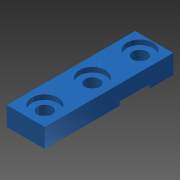
# Autodesk Inventor part: XCarriageBeltClampRight
Saved by Autodesk Inventor 2015 (Build 190159000, 159)
## iProperties
Created: 2014-08-22
Part Number: XCarriageBeltClampRight
Material: ABS Plastic
Document SubType Name: Modeling
Designer: t_clevj
Density: 1.06 g/cm^3
Appearance: Cyan
Author: t_clevj
Autodesk Inventor part; units mm, degrees
ref_plane "YZ Plane" through (0, 0, 0) normal (1, 0, 0) x (0, 1, 0)
ref_plane "XZ Plane" through (0, 0, 0) normal (0, 1, 0) x (-1, 0, 0)
ref_plane "XY Plane" through (0, 0, 0) normal (0, 0, 1) x (1, 0, 0)
sketch "Sketch1" plane through (0, 0, 0) normal (0, 0, 1) x (1, 0, 0)
  line L0 (0, 0) -> (8, 0)
  line L1 (8, 0) -> (8, 27)
  line L2 (8, 27) -> (0, 27)
  line L3 (0, 27) -> (0, 0)
  dimension "d0" = 27
  dimension "d1" = 8
  constraints: 8 end point, 2 parallel, 1 horizontal, 1 perpendicular
  measures "d0" distance of L2.end L0.start
  measures "d1" distance of L0.start L0.end
extrude "Extrusion1" add sketch "Sketch1" along normal blind 4
sketch "Sketch2" plane through (0, 0, 4) normal (0, 0, 1) x (1, 0, 0)
  line L0 (8, 0) -> (8, 27) projected
  line L1 (8, 27) -> (0, 27) projected
  point P0 (4, 24)
  point P1 (4, 14)
  point P2 (4, 4)
  dimension "d5" = 20
  dimension "d6" = 10
  dimension "d7" = 4
  dimension "d15" = 3
  constraints: 2 vertical alignment
  measures "d5" distance of point (4, 24) point (4, 4)
  measures "d6" distance of point (4, 4) point (4, 14)
  measures "d7" distance from line of L0 point (4, 4)
  measures "d15" distance from line of L1 point (4, 24)
hole "Hole1" at (4, 24, 4) at (4, 14, 4) at (4, 4, 4) direction (0, 0, -1) diameter 3 end up to face face through (2.6667, 18, 0) facing (0, 0, -1) counterbore diameter 5.5 counterbore depth 1
sketch "Sketch3" plane through (0, 0, 0) normal (0, 0, -1) x (-1, 0, 0)
  circle A0 centre (-4, 14) radius 1.5 projected
  line L0 (0, 27) -> (0, 0) projected
  line L1 (-8, 0) -> (-8, 27) projected
  line L2 (0, 27) -> (0, 0) construction
  line L3 (0, 22.25) -> (-8, 22.25) construction
  line L4 (-8, 0) -> (-8, 27) construction
  line L5 (-8, 15.75) -> (0, 15.75) construction
  line L6 (-8, 22.25) -> (-6.7, 22.25)
  line L7 (-6.7, 22.25) -> (-6.7, 15.75)
  line L8 (-6.7, 15.75) -> (-8, 15.75)
  line L9 (-8, 15.75) -> (-8, 22.25)
  line L10 (-6, 15.75) -> (-4.7, 15.75)
  line L11 (-4.7, 15.75) -> (-4.7, 22.25)
  line L12 (-4.7, 22.25) -> (-6, 22.25)
  line L13 (-6, 22.25) -> (-6, 15.75)
  line L14 (-4, 15.75) -> (-2.7, 15.75)
  line L15 (-2.7, 15.75) -> (-2.7, 22.25)
  line L16 (-2.7, 22.25) -> (-4, 22.25)
  line L17 (-4, 22.25) -> (-4, 15.75)
  line L18 (-2, 15.75) -> (-0.7, 15.75)
  line L19 (-0.7, 15.75) -> (-0.7, 22.25)
  line L20 (-0.7, 22.25) -> (-2, 22.25)
  line L21 (-2, 22.25) -> (-2, 15.75)
  dimension "d16" = 6.5
  dimension "d17" = 1.75
  dimension "d18" = 1.3
  dimension "d19" = 1.3
  dimension "d20" = 0.7
  dimension "d21" = 1.3
  dimension "d22" = 0.7
  dimension "d23" = 1.3
  dimension "d24" = 0.7
  constraints: 36 end point, 10 point on line, 8 parallel, 6 perpendicular, 4 horizontal, 1 midpoint
  measures "d16" distance between parallel lines of L3 L5
  measures "d17" distance from line of A0.centre L5
  measures "d18" distance between parallel lines of L1 L7
  measures "d19" distance between parallel lines of L13 L11
  measures "d20" distance between parallel lines of L7 L13
  measures "d21" distance between parallel lines of L15 L17
  measures "d22" distance between parallel lines of L11 L17
  measures "d23" distance between parallel lines of L21 L19
  measures "d24" distance between parallel lines of L15 L21
extrude "Extrusion2" cut sketch "Sketch3" against normal blind 0.8 contours L1 L6 L7 L8 | L13 L12 L11 L10 | L17 L16 L15 L14 | L21 L20 L19 L18
body "Solid1"
